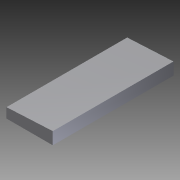
# Autodesk Inventor part: Fender
Saved by Autodesk Inventor 2012 (Build 160160000, 160)
## iProperties
Created: 2012-01-07
Part Number: Fender
Material: Default
Document SubType Name: Modeling
Designer: Justin
Density: 1 g/cm^3
Author: Justin
Autodesk Inventor part; units mm, degrees
ref_plane "YZ Plane" through (0, 0, 0) normal (1, 0, 0) x (0, 1, 0)
ref_plane "XZ Plane" through (0, 0, 0) normal (0, 1, 0) x (-1, 0, 0)
ref_plane "XY Plane" through (0, 0, 0) normal (0, 0, 1) x (1, 0, 0)
sketch "Sketch1" plane through (0, 0, 0) normal (0, 0, 1) x (1, 0, 0)
  line L0 (0, 0) -> (0, 209.55)
  line L1 (0, 209.55) -> (984.25, 260.35)
  line L2 (984.25, 260.35) -> (984.25, 0)
  line L3 (984.25, 0) -> (0, 0)
  dimension "d2" = 984.25
  dimension "d3" = 209.55
  dimension "d4" = 260.35
  constraints: 8 end point, 1 parallel, 1 perpendicular, 1 vertical
  measures "d2" distance of L2.end L0.start
  measures "d3" distance of L0.start L0.end
  measures "d4" distance of L1.end L2.end
extrude "Extrusion1" add sketch "Sketch1" along normal blind 2565.4
body "Solid1"
